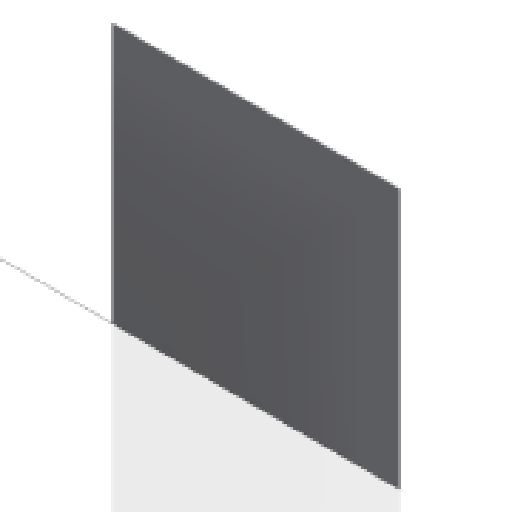
# Autodesk Inventor part: Rear Panel
Saved by Autodesk Inventor 2023.2 (Build 272271000, 271)
## iProperties
Created: 2023-02-06
Part Number: Rear Panel
Material: Aluminum 6061
Document SubType Name: Modeling
Designer: remop
Density: 2.7 g/cm^3
Appearance: Aluminum - Flat
Author: remop
Autodesk Inventor part; units mm, degrees
ref_plane "YZ Plane" through (0, 0, 0) normal (1, 0, 0) x (0, 1, 0)
ref_plane "XZ Plane" through (0, 0, 0) normal (0, 1, 0) x (-1, 0, 0)
ref_plane "XY Plane" through (0, 0, 0) normal (0, 0, 1) x (1, 0, 0)
sketch "Sketch1" plane through (0, 0, 0) normal (0, 0, 1) x (1, 0, 0)
  line L0 (287.336, -253.0124) -> (287.336, 226.9876) projected
  line L1 (287.336, 226.9876) -> (289.336, 226.9876) projected
  line L2 (289.336, -253.0124) -> (289.336, 226.9876) projected
  line L3 (287.336, -253.0124) -> (289.336, -253.0124) projected
  line L4 (-242.664, 226.9876) -> (-242.664, -253.0124) projected
  line L5 (-242.664, -253.0124) -> (-244.664, -253.0124) projected
  line L6 (-244.664, 226.9876) -> (-244.664, -253.0124) projected
  line L7 (-242.664, 226.9876) -> (-244.664, 226.9876) projected
  line L8 (287.336, 226.9876) -> (-242.664, 226.9876)
  line L9 (-242.664, -253.0124) -> (287.336, -253.0124)
  circle A0 centre (187.336, 219.4876) radius 1.75
  circle A1 centre (-142.664, 219.4876) radius 1.75
  circle A2 centre (22.336, 219.4876) radius 1.75
  circle A3 centre (187.336, -245.5124) radius 1.75
  circle A4 centre (22.336, -245.5124) radius 1.75
  circle A5 centre (-142.664, -245.5124) radius 1.75
  circle A6 centre (279.836, 161.9876) radius 1.75
  circle A7 centre (279.836, -188.0124) radius 1.75
  circle A8 centre (-235.164, -188.0124) radius 1.75
  circle A9 centre (-235.164, 161.9876) radius 1.75
  point P0 (0, 0)
  point P1 (22.336, 226.9876)
  dimension "d0" = 7.5
  dimension "d1" = 100
  dimension "d2" = 100
  dimension "d3" = 3.5
  dimension "d4" = 7.5
  dimension "d7" = 65
  dimension "d8" = 65
  dimension "d10" = 7.5
  dimension "d11" = 7.5
  constraints: 10 centre point, 9 equal radius, 6 horizontal alignment, 6 vertical alignment, 4 end point, 1 horizontal, 1 midpoint, 1 parallel
  measures "d0" distance from line of A0.centre L8
  measures "d1" distance from line of L0 A0.centre
  measures "d2" distance from line of L4 A1.centre
  measures "d3" diameter of A2
  measures "d4" distance from line of L9 A3.centre
  measures "d7" distance from line of A7.centre L9
  measures "d8" distance from line of L8 A6.centre
  measures "d10" distance from line of L4 A9.centre
  measures "d11" distance from line of L0 A6.centre
extrude "Extrusion1" add sketch "Sketch1" against normal blind 2
equation "\"d2\" = d1"
equation "\"d8\" = d7"
equation "\"d10\" = d9"
equation "\"d11\" = d4"
equation "\"d9\" = d4"
body "Solid1"
